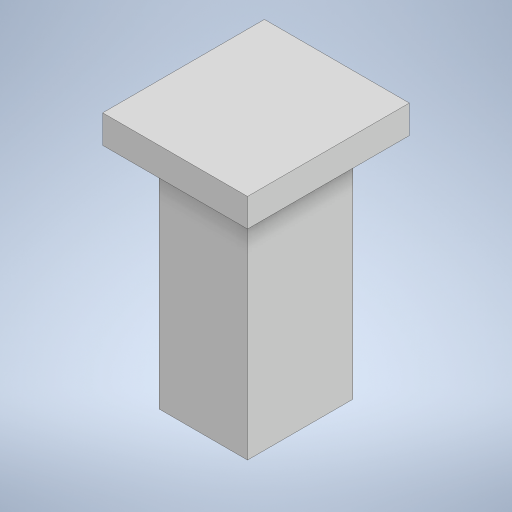
# Autodesk Inventor part: chaveta
Saved by Autodesk Inventor 2023 (Build 270158000, 158)
## iProperties
Created: 2024-08-19
Part Number: chaveta
Material: Generic
Document SubType Name: Modeling
Designer: sebas
Density: 1 g/cm^3
Appearance: Default
Author: sebas
Autodesk Inventor part; units mm, degrees
ref_plane "YZ Plane" through (0, 0, 0) normal (1, 0, 0) x (0, 1, 0)
ref_plane "XZ Plane" through (0, 0, 0) normal (0, 1, 0) x (-1, 0, 0)
ref_plane "XY Plane" through (0, 0, 0) normal (0, 0, 1) x (1, 0, 0)
sketch "Sketch1" plane through (0, 0, 0) normal (0, 1, 0) x (-1, 0, 0)
  line L0 (0, 0) -> (0, -18.7)
  line L1 (0, -18.7) -> (0, -11.8708)
  line L2 (0, -18.7) -> (15.7, -18.7)
  line L3 (15.7, -18.7) -> (15.7, 0)
  line L4 (15.7, 0) -> (0, 0)
  dimension "d0" = 18.7
  dimension "d1" = 15.7
  constraints: 10 end point, 3 perpendicular, 1 point on line, 1 vertical
  measures "d0" distance of L0.start L0.end
  measures "d1" distance of L0.end L2.end
extrude "Extrusion1" add sketch "Sketch1" along normal blind 40.5
sketch "Sketch2" plane through (0, 40.5, 0) normal (0, 1, 0) x (1, 0, 0)
  line L0 (0, 0) -> (0, 18.7) projected
  line L1 (0, 18.7) -> (0, 23.7)
  line L2 (0, 23.7) -> (-15.7, 23.7)
  line L3 (-15.7, 23.7) -> (-20.7, 23.7)
  line L4 (-20.7, 23.7) -> (-20.7, 0)
  line L5 (-20.7, 0) -> (-20.7, -5)
  line L6 (-20.7, -5) -> (0, -5)
  line L7 (0, -5) -> (5, -5)
  line L8 (5, -5) -> (5, 18.7)
  line L9 (5, 18.7) -> (5, 23.7)
  line L10 (0, 23.7) -> (5, 23.7)
  dimension "d4" = 5
  dimension "d5" = 5
  dimension "d6" = 5
  dimension "d7" = 5
  constraints: 20 end point, 6 point on line, 5 perpendicular, 1 vertical
  measures "d4" distance of L0.end L1.end
  measures "d5" distance of L2.end L3.end
  measures "d6" distance of L4.end L5.end
  measures "d7" distance of L6.end L7.end
extrude "Extrusion2" add sketch "Sketch2" along normal blind 5
body "Solid1"
